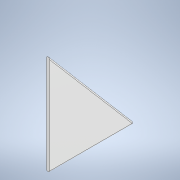
# Autodesk Inventor part: RedSail-ver1-1111-2021
Saved by Autodesk Inventor 2021 (Build 250183000, 183)
## iProperties
Created: 2021-03-03
Part Number: RedSail-ver1-1111-2021
Material: Generic
Document SubType Name: Modeling
Designer: CMurray
Density: 1 g/cm^3
Appearance: Fine Textured - White
Author: CMurray
Autodesk Inventor part; units mm, degrees
ref_plane "XZ Plane" through (0, 0, 0) normal (0, 1, 0) x (-1, 0, 0)
ref_plane "XY Plane" through (0, 0, 0) normal (0, 0, 1) x (1, 0, 0)
sketch "Sketch1" plane through (0, 0, 0) normal (1, 0, 0) x (0, 1, 0)
  line L0 (0, 0) -> (0, -1828.8)
  line L1 (0, -1828.8) -> (2133.6, 0)
  line L2 (2133.6, 0) -> (0, 0)
  dimension "d2" = 1828.8
  dimension "d3" = 2133.6
  constraints: 6 end point, 1 perpendicular, 1 vertical
  measures "d2" distance of L0.start L0.end
  measures "d3" distance of L1.end L0.start
extrude "Extrusion1" add sketch "Sketch1" along normal blind 63.5
ref_plane "Work Plane1" through (31.75, 0, 0) normal (1, 0, 0) x (0, 1, 0)
fillet "Fillet4" radius 25.4 1 edges at (63.5, 1066.8, -914.4)
fillet "Fillet5" radius 25.4 1 edges at (0, 1066.8, -914.4)
fillet "Fillet6" radius 25.4 5 edges at (56.0605, 0, -1819.0016) (31.75, 0, -1828.8) (7.4395, 0, -1819.0016) (0, 0, -897.6731) (63.5, 0, -897.6731)
body "Solid1"
